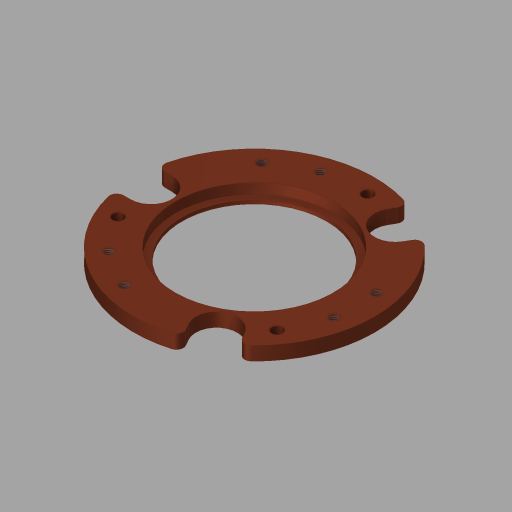
# Autodesk Inventor part: MiddleRing-2023-1
Saved by Autodesk Inventor 2024.2 (Build 282272000, 272)
## iProperties
Created: 2018-11-20
Part Number: MiddleRing-2023-1
Material: Copper
Document SubType Name: Modeling
Designer: schanen
Density: 8.94 g/cm^3
Appearance: Copper - Satin
Mass: 78.558 g
Surface Area: 62.0611 cm^2
Volume: 8.78725 cm^3
Author: schanen
Autodesk Inventor part; units mm, degrees
ref_plane "YZ Plane" through (0, 0, 0) normal (1, 0, 0) x (0, 1, 0)
ref_plane "XZ Plane" through (0, 0, 0) normal (0, 1, 0) x (-1, 0, 0)
ref_plane "XY Plane" through (0, 0, 0) normal (0, 0, 1) x (1, 0, 0)
sketch "Sketch1" plane through (0, 0, 0) normal (1, 0, 0) x (0, 1, 0)
  line L0 (0, 35) -> (4, 35)
  line L1 (4, 35) -> (4, 23)
  line L2 (1, 21) -> (0, 21)
  line L3 (0, 21) -> (0, 35)
  line L4 (-0.8, 0) -> (4.8, 0) projected
  line L5 (1, 23) -> (1, 21)
  line L6 (4, 23) -> (1, 23)
  point P0 (0, 0)
  dimension "d0" = 21
  dimension "d2" = 35
  dimension "d51" = 4
  dimension "d52" = 3
  dimension "d53" = 23
  constraints: 12 end point, 4 perpendicular, 2 horizontal, 1 point on line
  measures "d0" distance between parallel lines of L4 L2
  measures "d2" distance between parallel lines of L4 L0
  measures "d51" distance between parallel lines of L3 L1
  measures "d52" distance of L1.end L5.start
  measures "d53" distance between parallel lines of L4 L6
revolve "Revolution1" add sketch "Sketch1" angle 360 about axis through (0, -10, 0) along (0, 1, 0)
sketch "Sketch2" plane through (0, 4, 0) normal (0, 1, 0) x (1, 0, 0)
  arc A0 (-30, -6) -> (-30, 6) centre (-30, 0) ccw
  line L0 (-30, -6) -> (-34.4819, -6)
  circle A1 centre (0, 0) radius 35 projected
  line L1 (-30, 6) -> (-34.4819, 6)
  arc A2 (-34.4819, 6) -> (-34.4819, -6) centre (0, 0) ccw
  dimension "d6" = 12
  dimension "d7" = 30
  constraints: 6 point on circle, 4 end point, 2 centre point, 2 horizontal, 1 coincident, 1 tangent
  measures "d6" diameter of A0
  measures "d7" distance of point (0, 0) A0.centre
extrude "Extrusion1" cut sketch "Sketch2" against normal blind 4 contours L0 A1 L1 A0 picked at (-31.3095, 0.2411)
pattern_circular "Circular Pattern1" count 3 over 360 about axis through (0, 0.5, 0) along (0, 1, 0) of "Extrusion1"
sketch "Sketch3" plane through (-34.4819, 4, -6) normal (0, 1, 0) x (1, 0, 0)
  point P0 (34.4819, -6)
sketch "Sketch4" plane through (-34.4819, 4, -6) normal (0, 1, 0) x (1, 0, 0)
  circle A0 centre (34.4819, -6) radius 30 construction
  arc A1 (4.4819, -12) -> (4.4819, 0) centre (4.4819, -6) ccw projected
  point P0 (7.0755, -18.2021)
  dimension "d13" = 60
  dimension "d14" = 24
  constraints: 1 coincident, 3 other
hole "Hole1" at (-27.4064, 4, 12.2021) direction (0, -1, 0) diameter 3.2 end through all
pattern_circular "Circular Pattern2" count 3 over 360 about axis through (0, 0.5, 0) along (0, 1, 0) of "Hole1"
sketch "Sketch5" plane through (-34.4819, 4, -6) normal (0, 1, 0) x (1, 0, 0)
  circle A0 centre (34.4819, -6) radius 30 construction
  arc A1 (4.4819, -12) -> (4.4819, 0) centre (4.4819, -6) ccw projected
  point P0 (14.408, 16.2943)
  dimension "d25" = 60
  dimension "d26" = 48
  constraints: 1 coincident, 3 other
hole "Hole2" at (-20.0739, 4, -22.2943) direction (0, -1, 0) diameter 2.6211 end through all thread size "M3x0.35" class "6H" standard "ANSI Metric M Profile"
pattern_circular "Circular Pattern3" count 3 over 360 about axis through (0, 0.5, 0) along (0, 1, 0) of "Hole2"
sketch "Sketch6" plane through (-34.4819, 4, -6) normal (0, 1, 0) x (1, 0, 0)
  circle A0 centre (7.0755, -18.2021) radius 1.6 projected
  line L0 (34.4819, -6) -> (7.0755, -18.2021) construction
  circle A1 centre (34.4819, -6) radius 21 projected
  circle A2 centre (25.2114, -34.5317) radius 1.3106 projected
  line L1 (34.4819, -6) -> (25.2114, -34.5317) construction
  circle A3 centre (34.4819, -6) radius 30 construction
  point P0 (14.408, -28.2943)
  dimension "d37" = 60
  dimension "d38" = 48
  dimension "d39" = 24
  constraints: 4 end point, 1 coincident, 3 other
  measures "d38" angle of L1 L0
hole "Hole3" at (-20.0739, 4, 22.2943) direction (0, -1, 0) diameter 2.459 end through all thread size "M3x0.5" class "6H" standard "ANSI Metric M Profile"
pattern_circular "Circular Pattern4" count 3 over 360 about axis through (0, 0.5, 0) along (0, 1, 0) of "Hole3"
fillet "Fillet1" radius 2 6 edges at (12.0448, 2, 32.8622) (22.4371, 2, 26.8622) (22.4371, 2, -26.8622) (12.0448, 2, -32.8622) (-34.4819, 2, -6) (-34.4819, 2, 6)
equation "\"d39\" = 0.5 * d38"
body "Solid1"
